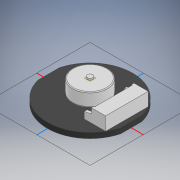
# Autodesk Inventor part: encoder
Saved by Autodesk Inventor 2022 (Build 260153000, 153)
## iProperties
Created: 2022-11-07
Part Number: encoder
Material: Типовые
Document SubType Name: Modeling
Designer: Petrov Ivan
Density: 1 g/cm^3
Appearance: По умолчанию
Author: Petrov Ivan
Autodesk Inventor part; units mm, degrees
ref_plane "YZ Plane" through (0, 0, 0) normal (1, 0, 0) x (0, 1, 0)
ref_plane "XZ Plane" through (0, 0, 0) normal (0, 1, 0) x (-1, 0, 0)
ref_plane "XY Plane" through (0, 0, 0) normal (0, 0, 1) x (1, 0, 0)
sketch "Эскиз1" plane through (0, 0, 0) normal (0, 1, 0) x (-1, 0, 0)
  circle A0 centre (0, 0) radius 16
  line L0 (15.5, 3.9686) -> (15.5, -3.9686)
  line L1 (-15.5, 3.9686) -> (-15.5, -3.9686)
  dimension "d0" = 32
  dimension "d1" = 15.5
  dimension "d2" = 15.5
  constraints: 4 end point, 4 point on circle, 1 centre point, 1 coincident, 1 parallel, 1 vertical
  measures "d0" diameter of A0
  measures "d1" distance from line of point (0, 0) L0
  measures "d2" distance from line of L1 point (0, 0)
extrude "Выдавливание1" add sketch "Эскиз1" along normal blind 2 contours L0 A0 L1
sketch "Эскиз2" plane through (0, 2, 0) normal (0, 1, 0) x (1, 0, 0)
  circle A0 centre (0, 0) radius 1
  dimension "d5" = 2
  constraints: 1 centre point, 1 coincident
  measures "d5" diameter of A0
extrude "Выдавливание2" add sketch "Эскиз2" along normal blind 7
ref_plane "РабПлоскость1" through (0, 8.4, 0) normal (0, 1, 0) x (1, 0, 0)
sketch "Эскиз3" plane through (0, 8.4, 0) normal (0, 1, 0) x (1, 0, 0)
  circle A0 centre (0, 0) radius 1 projected
  circle A1 centre (0, 0) radius 6.5
  dimension "d9" = 13
  constraints: 1 centre point, 1 coincident
  measures "d9" diameter of A1
extrude "Выдавливание3" add sketch "Эскиз3" against normal blind 5
fillet "Сопряжение1" radius 0.3 2 edges at (-6.5, 8.4, 0) (-6.5, 3.4, 0)
sketch "Эскиз4" plane through (0, 2, 0) normal (0, 1, 0) x (1, 0, 0)
  line L0 (13.8564, -8) -> (5.8564, -8)
  line L1 (5.8564, -8) -> (5.8564, 8)
  line L2 (5.8564, 8) -> (13.8564, 8)
  line L3 (13.8564, 8) -> (13.8564, -8)
  arc A0 (-15.5, -3.9686) -> (15.5, -3.9686) centre (0, 0) ccw projected
  arc A1 (15.5, 3.9686) -> (-15.5, 3.9686) centre (0, 0) ccw projected
  line L4 (5.8564, -7) -> (8.8564, -7)
  line L5 (8.8564, -7) -> (8.8564, 7)
  line L6 (8.8564, 7) -> (5.8564, 7)
  line L7 (5.8564, 7) -> (5.8564, -7)
  line L8 (13.8564, 0) -> (12.4148, 0) construction
  dimension "d13" = 8
  dimension "d14" = 16
  dimension "d21" = 5
  dimension "d22" = 14
  constraints: 18 end point, 4 parallel, 3 horizontal, 2 perpendicular, 2 point on circle, 1 midpoint, 1 point on line, 1 other
  measures "d13" distance of L1.end L2.end
  measures "d14" distance of L0.end L1.end
  measures "d21" distance between parallel lines of L3 L5
  measures "d22" distance of L4.end L5.end
extrude "Выдавливание4" add sketch "Эскиз4" along normal blind 5 contours L0 L1 L4 L5 L6 L2 L3
sketch "Эскиз6" plane through (5.8564, 2, 8) normal (0, 0, 1) x (1, 0, 0)
  line L0 (0, 0) -> (0, 5) projected
  line L1 (0, 0) -> (0, 2.5)
  line L2 (0, 2.5) -> (2.6743, 3)
  line L3 (2.6743, 3) -> (2.6743, 5)
  line L4 (8, 5) -> (0, 5) projected
  point P0 (-5.8564, -2)
  dimension "d23" = 2.5
  dimension "d24" = 2
  constraints: 6 end point, 1 midpoint, 1 parallel, 1 point on line
  measures "d23" distance of L0.start L1.end
  measures "d24" distance of L2.end L3.end
extrude "Выдавливание6" cut sketch "Эскиз6" against normal blind 5
mirror "Зеркальное отражение1" about plane through (0, 0, 0) normal (0, 0, 1) of "Выдавливание6"
equation "\"d2\" = d1"
